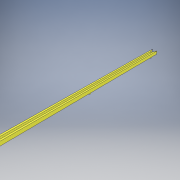
# Autodesk Inventor part: CardGuide-2#01
Saved by Autodesk Inventor 2018 (Build 220112000, 112)
## iProperties
Created: 2025-02-16
Part Number: CardGuide-2#01
Material: Všeobecné
Document SubType Name: Modeling
Designer: Jozko Mrkvicka
Density: 1 g/cm^3
Appearance: Výchozí
Author: Jozko Mrkvicka
Autodesk Inventor part; units mm, degrees
ref_plane "YZ Plane" through (0, 0, 0) normal (1, 0, 0) x (0, 1, 0)
ref_plane "XZ Plane" through (0, 0, 0) normal (0, 1, 0) x (-1, 0, 0)
ref_plane "XY Plane" through (0, 0, 0) normal (0, 0, 1) x (1, 0, 0)
sketch "Náčrt1" plane through (0, 0, 0) normal (0, 1, 0) x (-1, 0, 0)
  line L0 (0, 0) -> (6.35, 0)
  line L1 (6.35, 0) -> (6.35, -215.9)
  line L2 (6.35, -215.9) -> (0, -215.9)
  line L3 (0, -215.9) -> (0, 0)
  dimension "d0" = 215.9
  dimension "d1" = 6.35
  constraints: 8 end point, 2 parallel, 1 horizontal, 1 perpendicular
  measures "d0" distance of L0.end L1.end
  measures "d1" distance of L0.start L0.end
extrude "Vysunutí1" add sketch "Náčrt1" along normal blind 1.27
sketch "Náčrt2" plane through (0, 1.27, 0) normal (0, 1, 0) x (1, 0, 0)
  line L0 (-1.905, 5.4741) -> (-1.905, 210.4259)
  line L1 (-4.445, 210.4259) -> (-4.445, 5.4741)
  line L2 (-6.35, 0) -> (-4.445, 5.4741)
  line L3 (0, 0) -> (-1.905, 5.4741)
  line L4 (-6.35, 215.9) -> (-4.445, 210.4259)
  line L5 (-6.35, 215.9) -> (-6.35, 0) projected
  line L6 (-6.35, 0) -> (-6.35, 215.9)
  line L7 (0, 215.9) -> (0, 0)
  line L8 (0, 215.9) -> (-6.35, 215.9) projected
  line L9 (-1.905, 210.4259) -> (0, 215.9)
  dimension "d29" = 19.188
  dimension "d30" = 19.188
  dimension "d34" = 2.54
  constraints: 16 end point, 5 equal length, 2 vertical
  measures "d29" angle of L5 L2
  measures "d30" angle of L7 L3
  measures "d34" distance between parallel lines of L0 L1
chamfer "Zkosení1" distance 5.588 distance2 1.27 1 edges at (-3.175, 1.27, 0) measured on face at (-3.175, 1.27, -0.5)
chamfer "Zkosení2" distance 5.588 distance2 1.27 1 edges at (-3.175, 1.27, -215.9) measured on face at (-3.175, 1.27, -215.4)
extrude "Vysunutí3" add sketch "Náčrt2" along normal blind 3.175 and the other way blind 1.27
sketch "Náčrt4" plane through (0, 0, 0) normal (0, -1, 0) x (1, 0, 0)
  line L0 (-1.905, -5.588) -> (-4.445, -5.588) projected
  circle A0 centre (-3.175, -5.588) radius 1.5
  point P0 (-2.2098, -6.35)
  point P1 (-4.1402, -6.35)
  point P2 (-1.8562, -5.334)
  point P3 (-4.4938, -5.334)
  dimension "d26" = 3
  constraints: 1 centre point, 2 other
  measures "d26" diameter of A0
extrude "Vysunutí4" add sketch "Náčrt4" along normal blind 3.175
pattern_linear "Obdélníkové pole1" count 3 spacing 101.6 along (0, 0, -1) of "Vysunutí4"
fillet "Zaoblení2" radius 0.254 3 edges at (-4.675, -3.175, -5.588) (-4.675, -3.175, -107.188) (-4.675, -3.175, -208.788)
equation "\"d0\" = length"
equation "\"d34\" = gPcbThickness"
equation "\"d37\" = pinDistance"
equation "\"length\" = 215.9"
equation "\"pinDistance\" = 101.6"
equation "\"gPcbThickness\" = 2.54"
